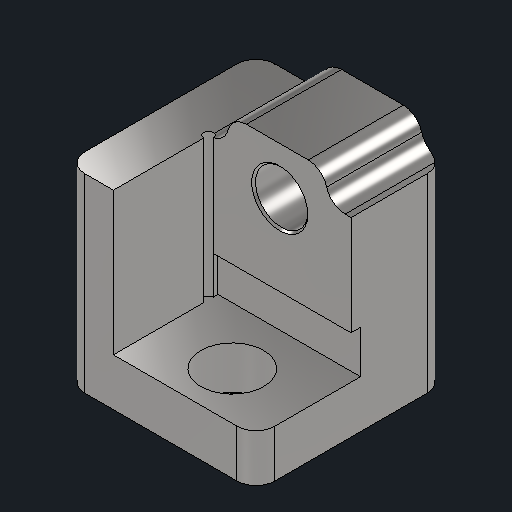
# Autodesk Inventor part: KN-00-02-08
Saved by Autodesk Inventor 2025.2 (Build 292293000, 293)
## iProperties
Created: 2025-04-21
Part Number: KN-00-02-08
Material: X5CrNi18-10
Document SubType Name: Modeling
Designer: Kacper Mik
Density: 8 g/cm^3
Appearance: Semi-Polished
Mass: 44.1461 g
Surface Area: 26.2679 cm^2
Volume: 5.51827 cm^3
Author: Kacper Mik
Autodesk Inventor part; units mm, degrees
note: some values were not read from the file. Chosen so that the rebuilt part matches the saved one: direction of "Hole4".
ref_plane "YZ Plane" through (0, 0, 0) normal (1, 0, 0) x (0, 1, 0)
ref_plane "XZ Plane" through (0, 0, 0) normal (0, 1, 0) x (-1, 0, 0)
sketch "Sketch1" plane through (0, 0, 0) normal (0, 1, 0) x (-1, 0, 0)
  line L0 (0, 0) -> (20, 0)
  line L1 (20, 0) -> (20, -20)
  line L2 (20, -20) -> (0, -20)
  line L3 (0, -20) -> (0, 0)
  dimension "d0" = 20
  dimension "d1" = 20
  constraints: 8 end point, 2 parallel, 1 horizontal, 1 perpendicular
  measures "d0" distance of L1.end L2.end
  measures "d1" distance of L0.end L1.end
extrude "Extrusion1" add sketch "Sketch1" along normal blind 5
sketch "Sketch2" plane through (0, 5, 0) normal (0, 1, 0) x (1, 0, 0)
  line L0 (0, 0) -> (0, 20) projected
  line L1 (-20, 0) -> (0, 0) projected
  point P0 (-7.5, 5)
  dimension "d4" = 7.5
  dimension "d55" = 5
  measures "d4" distance from line of L0 point (-7.5, 5)
  measures "d55" distance from line of L1 point (-7.5, 5)
hole "Hole1" at (-7.5, 5, -5) direction (0, -1, 0) diameter 6.6 end through all clearance for "Countersunk Flat Head Screw ISO 2009/7046" size "M6" standard "ISO"
chamfer "Chamfer1" distance 0.5 angle 45 1 edges at (-7.5, 0, -8.3)
sketch "Sketch3" plane through (0, 5, 0) normal (0, 1, 0) x (1, 0, 0)
  circle A0 centre (-7.5, 5) radius 3.3 construction
  line L0 (0, 20) -> (-20, 20) construction
  line L1 (-20, 20) -> (-20, 0) construction
  line L2 (-20, 0) -> (0, 0) construction
  line L3 (0, 0) -> (0, 20) construction
  line L4 (-20, 20) -> (-20, 0) construction
  line L5 (0, 20) -> (-20, 20) construction
  line L6 (-20, 0) -> (-15, 0)
  line L7 (-15, 0) -> (-15, 20)
  line L8 (-15, 20) -> (-20, 20)
  line L9 (-20, 20) -> (-20, 0)
  line L10 (0, 20) -> (-20, 20)
  line L11 (-20, 20) -> (-20, 10)
  line L12 (-20, 10) -> (0, 10)
  line L13 (0, 10) -> (0, 20)
  point P0 (-15, 10)
  dimension "d56" = 15
  dimension "d57" = 10
  constraints: 16 end point, 4 parallel, 2 horizontal, 2 perpendicular, 1 midpoint, 1 point on line
  measures "d56" distance between parallel lines of L3 L7
  measures "d57" distance between parallel lines of L2 L12
extrude "Extrusion2" add sketch "Sketch3" along normal blind 15
sketch "Sketch6" plane through (0, 20, 0) normal (0, 1, 0) x (1, 0, 0)
  line L0 (0, 20) -> (-20, 20) construction
  line L1 (-20, 20) -> (-20, 0) construction
  line L2 (-20, 0) -> (-15, 0) construction
  line L3 (-15, 0) -> (-15, 10) construction
  line L4 (-15, 10) -> (0, 10) construction
  line L5 (0, 10) -> (0, 20) construction
  line L6 (-2.5, 10) -> (-13, 10)
  line L7 (-13, 10) -> (-13, 20)
  line L8 (-13, 20) -> (-2.5, 20)
  line L9 (-2.5, 20) -> (-2.5, 10)
  dimension "d32" = 2.5
  dimension "d33" = 10.5
  dimension "d34" = 2
  constraints: 8 end point, 2 parallel, 2 point on line, 1 horizontal, 1 perpendicular
  measures "d32" distance between parallel lines of L5 L9
  measures "d33" distance between parallel lines of L7 L9
  measures "d34" distance between parallel lines of L3 L7
extrude "Extrusion5" add sketch "Sketch6" along normal blind 3
fillet "Fillet4" radius 2 6 edges at (-13, 23, -15) (-2.5, 23, -15) (0, 2.5, 0) (-20, 10, 0) (0, 10, -20) (-20, 10, -20)
sketch "Sketch7" plane through (0, 5, -10) normal (0, 0, 1) x (1, 0, 0)
  line L0 (-11, 18) -> (-4.5, 18) projected
  line L1 (0, 0) -> (0, 15) projected
  point P0 (0, -5)
  point P1 (-7.5, 13)
  dimension "d36" = 5
  dimension "d58" = 7.5
  measures "d36" distance from line of L0 point (-7.5, 13)
  measures "d58" distance from line of L1 point (-7.5, 13)
hole "Hole2" at (-7.5, 18, -10) direction (0, 0, -1) diameter 5.5 end through all clearance for "Countersunk Flat Head Screw ISO 2009/7046" size "M5" standard "ISO"
fillet "Fillet5" radius 2 2 edges at (-2.5, 20, -15) (-13, 20, -15)
chamfer "Chamfer2" distance 0.2 angle 45 1 edges at (-7.5, 20.75, -10)
ref_plane "Work Plane1" through (0, 21, 0) normal (0, 1, 0) x (1, 0, 0)
sketch "Sketch9" plane through (0, 21, 0) normal (0, 1, 0) x (1, 0, 0)
  line L0 (-15, 10) -> (-15, 0) projected
  point P0 (0, 0)
hole "Hole4" at (-15, 21, -10) direction (0, -1, 0) diameter 1 depth 16
sketch "Sketch10" plane through (0, 5, -10) normal (1, 0, 0) x (0, 0, -1)
  line L0 (8, 15) -> (8, -5) construction
  line L1 (0, 15) -> (8, 15) construction
  line L2 (0, 0) -> (0, 15) construction
  line L3 (-8, 0) -> (0, 0) construction
  line L4 (-8, -5) -> (-8, 0) construction
  line L5 (-8, -5) -> (8, -5) construction
  line L6 (0, 0) -> (1, 0)
  line L7 (1, 0) -> (1, 4.5)
  line L8 (1, 4.5) -> (0, 4.5)
  line L9 (0, 4.5) -> (0, 0)
  point P0 (-10, -5)
  dimension "d67" = 1
  dimension "d68" = 4.5
  constraints: 8 end point, 2 parallel, 1 horizontal, 1 perpendicular
  measures "d67" distance of L8.end L7.end
  measures "d68" distance of L7.end L6.end
extrude "Extrusion6" cut sketch "Sketch10" against normal up to surface (15 mm away)
body "Solid1"
